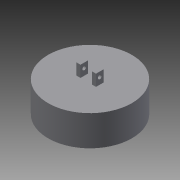
# Autodesk Inventor part: manipulator base
Saved by Autodesk Inventor 2015 (Build 190159000, 159)
## iProperties
Created: 2014-10-18
Part Number: manipulator base
Material: Generic
Document SubType Name: Modeling
Designer: ericd_000
Density: 1 g/cm^3
Appearance: Default
Author: ericd_000
Autodesk Inventor part; units mm, degrees
ref_plane "YZ Plane" through (0, 0, 0) normal (1, 0, 0) x (0, 1, 0)
ref_plane "XZ Plane" through (0, 0, 0) normal (0, 1, 0) x (-1, 0, 0)
ref_plane "XY Plane" through (0, 0, 0) normal (0, 0, 1) x (1, 0, 0)
sketch "Sketch1" plane through (0, 0, 0) normal (0, 0, 1) x (1, 0, 0)
  circle A0 centre (0, 0) radius 55
  dimension "d0" = 110
  constraints: 1 centre point, 1 coincident
  measures "d0" diameter of A0
extrude "Extrusion1" add sketch "Sketch1" along normal blind 40
sketch "Sketch2" plane through (0, 0, 40) normal (0, 0, 1) x (1, 0, 0)
  line L0 (-7.5, 0) -> (7.5, 0) construction
  line L1 (-12.8812, 5) -> (-7.5, 5)
  line L2 (-7.5, 5) -> (-7.5, -5)
  line L3 (-7.5, -5) -> (-12.8812, -5)
  line L4 (-12.8812, -5) -> (-12.8812, 5)
  line L5 (7.5, 5) -> (12.8812, 5)
  line L6 (12.8812, 5) -> (12.8812, -5)
  line L7 (12.8812, -5) -> (7.5, -5)
  line L8 (7.5, -5) -> (7.5, 5)
  point P0 (0, 0)
  point P1 (0, 0)
  dimension "d3" = 15
  dimension "d6" = 10
  dimension "d7" = 10
  constraints: 18 end point, 5 coincident, 4 parallel, 3 horizontal, 3 midpoint, 2 perpendicular
  measures "d3" distance of L0.start L0.end
  measures "d6" distance of L5.end L6.end
  measures "d7" distance of L3.end L1.start
extrude "Extrusion2" add sketch "Sketch2" along normal blind 15
sketch "Sketch3" plane through (-12.8812, -5, 40) normal (-1, 0, 0) x (0, 0, 1)
  circle A0 centre (8.6714, 5) radius 2.5
  line L0 (15, 10) -> (15, 0) projected
  point P0 (-40, 5)
  point P1 (15, 5)
  dimension "d8" = 5
  constraints: 1 centre point, 1 horizontal alignment, 1 midpoint
  measures "d8" diameter of A0
extrude "Extrusion3" cut sketch "Sketch3" against normal up to surface (25.7623 mm away)
body "Solid1"
